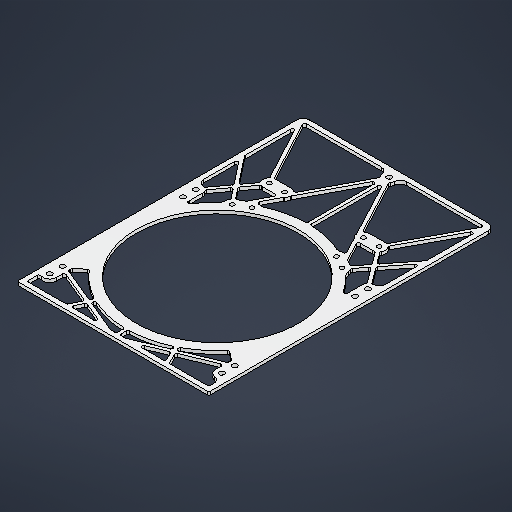
# Autodesk Inventor part: PLATE,SHOOTER,BOTTOM
Saved by Autodesk Inventor 2026.1 (Build 301233020, 233B)
## iProperties
Created: 2026-01-27
Part Number: PLATE,SHOOTER,BOTTOM
Material: Aluminum 6061
Document SubType Name: Sheet Metal
Designer: Owen L
Density: 2.7 g/cm^3
Appearance: Aluminum - Flat
Mass: 268.69 g
Surface Area: 679.811 cm^2
Volume: 99.5147 cm^3
Sheet Metal Rule: Default
Author: Owen L
Autodesk Inventor part; units mm, degrees
ref_plane "YZ Plane" through (0, 0, 0) normal (1, 0, 0) x (0, 1, 0)
ref_plane "XZ Plane" through (0, 0, 0) normal (0, 1, 0) x (-1, 0, 0)
ref_plane "XY Plane" through (0, 0, 0) normal (0, 0, 1) x (1, 0, 0)
sketch "Sketch1" plane through (0, 0, 0) normal (0, 1, 0) x (-1, 0, 0)
  line L0 (-93.6625, 139.7) -> (93.6625, 139.7)
  line L1 (93.6625, 139.7) -> (93.6625, -139.7)
  line L2 (93.6625, -139.7) -> (-93.6625, -139.7)
  line L3 (-93.6625, -139.7) -> (-93.6625, 139.7)
  line L4 (-93.6625, 139.7) -> (93.6625, -139.7) construction
  line L5 (93.6625, 139.7) -> (-93.6625, -139.7) construction
  circle A0 centre (0, 37.7949) radius 79.375
  point P0 (0, 0)
  dimension "d0" = 187.325
  dimension "d1" = 279.4
  dimension "d2" = 158.75
  dimension "d3" = 101.9051
  measures "d0" distance of L1.end L2.end
  measures "d1" distance of L0.end L1.end
  measures "d2" diameter of A0
  measures "d3" distance from line of L0 A0.centre
extrude "Plate1" add sketch "Sketch1" along normal blind 3.175
fillet "Corner Round1" radius 6.35 2 edges at (-93.6625, 1.5875, -139.7) (93.6625, 1.5875, -139.7)
fillet "Corner Round1" radius 1.5875 2 edges at (-93.6625, 1.5875, 139.7) (93.6625, 1.5875, 139.7)
sketch "Sketch2" plane through (0, 0, 0) normal (0, -1, 0) x (1, 0, 0)
  point P0 (0, 0)
  point P1 (-41.275, -37.3842)
  point P2 (-38.4175, -66.5942)
  point P3 (-53.6575, -66.5942)
  point P4 (-53.6575, -30.3992)
  dimension "d7" = 37.3842
  dimension "d11" = 41.275
  dimension "d12" = 6.985
  dimension "d13" = 29.21
  dimension "d14" = 2.8575
  dimension "d15" = 12.3825
  constraints: 1 horizontal alignment, 1 vertical alignment
  measures "d7" vertical distance of point (-41.275, -37.384) point (0, 0)
  measures "d11" horizontal distance of point (0, 0) point (-41.275, -37.384)
  measures "d12" vertical distance of point (-53.658, -30.399) point (-41.275, -37.384)
  measures "d13" vertical distance of point (-38.418, -66.594) point (-41.275, -37.384)
  measures "d14" horizontal distance of point (-38.418, -66.594) point (-41.275, -37.384)
  measures "d15" horizontal distance of point (-53.658, -66.594) point (-41.275, -37.384)
hole "Hole1" at (-41.275, 0, -37.3842) at (-38.4175, 0, -66.5942) at (-53.6575, 0, -66.5942) at (-53.6575, 0, -30.3992) direction (0, 1, 0) diameter 4.2926 depth 3.175 clearance for "Flat Head Machine Screw" size "M4" standard "Ansi Metric M Profile"
mirror "Mirror1" about plane through (0, 0, 0) normal (1, 0, 0) of "Hole1"
sketch "Sketch3" plane through (0, 3.175, 0) normal (0, 1, 0) x (1, 0, 0)
  line L0 (93.6625, -139.7) -> (-93.6625, -139.7) construction
  line L1 (93.6625, 133.35) -> (93.6625, -139.7) construction
  line L2 (-87.3125, 139.7) -> (87.3125, 139.7) construction
  line L3 (0, -139.7) -> (0, 139.7) construction
  point P0 (0, 0)
  point P1 (84.1375, -117.475)
  point P2 (84.1375, -104.775)
  point P3 (84.1375, 12.7)
  point P4 (84.1375, 25.4)
  point P5 (0, 130.175)
  point P6 (-84.1375, -117.475)
  point P7 (-84.1375, -104.775)
  point P8 (-84.1375, 12.7)
  point P9 (-84.1375, 25.4)
  dimension "d23" = 22.225
  dimension "d24" = 12.7
  dimension "d25" = 9.525
  dimension "d26" = 12.7
  dimension "d27" = 107.95
  dimension "d28" = 9.525
  constraints: 4 symmetric about line, 4 vertical alignment, 2 end point, 2 midpoint
  measures "d23" distance from line of L0 point (84.138, -117.475)
  measures "d24" distance of point (84.138, -104.775) point (84.138, -117.475)
  measures "d25" distance from line of L1 point (84.138, -117.475)
  measures "d26" distance of point (84.138, 25.4) point (84.138, 12.7)
  measures "d27" vertical distance of L1.start point (84.138, 25.4)
  measures "d28" distance from line of L2 point (0, 130.175)
hole "Hole2" at (84.1375, 3.175, 117.475) at (84.1375, 3.175, 104.775) at (84.1375, 3.175, -12.7) at (84.1375, 3.175, -25.4) at (0, 3.175, -130.175) at (-84.1375, 3.175, -25.4) at (-84.1375, 3.175, -12.7) at (-84.1375, 3.175, 104.775) at (-84.1375, 3.175, 117.475) direction (0, -1, 0) diameter 4.9784 depth 3.175 clearance for "Flat Head Machine Screw (82)" size "#10" standard "Ansi Unified Screw Threads"
sketch "Sketch4" plane through (0, 0, 0) normal (0, -1, 0) x (1, 0, 0)
  circle A0 centre (-84.1375, 117.475) radius 2.4892 projected
  circle A1 centre (-84.1375, 104.775) radius 2.4892 projected
  circle A2 centre (-84.1375, -12.7) radius 2.4892 projected
  circle A3 centre (-84.1375, -25.4) radius 2.4892 projected
  circle A4 centre (0, -130.175) radius 2.4892 projected
  circle A5 centre (84.1375, -25.4) radius 2.4892 projected
  circle A6 centre (84.1375, -12.7) radius 2.4892 projected
  circle A7 centre (84.1375, 104.775) radius 2.4892 projected
  circle A8 centre (84.1375, 117.475) radius 2.4892 projected
  circle A9 centre (53.6575, -30.3992) radius 2.1463 projected
  circle A10 centre (53.6575, -66.5942) radius 2.1463 projected
  circle A11 centre (38.4175, -66.5942) radius 2.1463 projected
  circle A12 centre (41.275, -37.3842) radius 2.1463 projected
  circle A13 centre (-53.6575, -30.3992) radius 2.1463 projected
  circle A14 centre (-53.6575, -66.5942) radius 2.1463 projected
  circle A15 centre (-38.4175, -66.5942) radius 2.1463 projected
  circle A16 centre (-41.275, -37.3842) radius 2.1463 projected
  circle A17 centre (0, 37.7949) radius 79.375 projected
  arc A18 (93.6625, 138.1125) -> (92.075, 139.7) centre (92.075, 138.1125) ccw projected
  line L0 (-92.075, 139.7) -> (92.075, 139.7) projected
  arc A19 (-92.075, 139.7) -> (-93.6625, 138.1125) centre (-92.075, 138.1125) ccw projected
  line L1 (-93.6625, -133.35) -> (-93.6625, 138.1125) projected
  arc A20 (-93.6625, -133.35) -> (-87.3125, -139.7) centre (-87.3125, -133.35) ccw projected
  line L2 (87.3125, -139.7) -> (-87.3125, -139.7) projected
  arc A21 (87.3125, -139.7) -> (93.6625, -133.35) centre (87.3125, -133.35) ccw projected
  line L3 (93.6625, 138.1125) -> (93.6625, -133.35) projected
  line L4 (-88.9, 134.9375) -> (88.9, 134.9375)
  line L5 (88.9, 134.9375) -> (88.9, -133.35)
  arc A22 (87.3125, -134.9375) -> (88.9, -133.35) centre (87.3125, -133.35) ccw
  line L6 (87.3125, -134.9375) -> (-87.3125, -134.9375)
  arc A23 (-88.9, -133.35) -> (-87.3125, -134.9375) centre (-87.3125, -133.35) ccw
  line L7 (-88.9, -133.35) -> (-88.9, 134.9375)
  circle A24 centre (0, 37.7949) radius 88.9
  circle A25 centre (0, -130.175) radius 6.35
  circle A26 centre (-84.1375, -25.4) radius 2.4892 projected
  circle A27 centre (-84.1375, -25.4) radius 6.35
  circle A28 centre (-84.1375, -12.7) radius 6.35
  circle A29 centre (-84.1375, 104.775) radius 6.35
  circle A30 centre (-84.1375, 117.475) radius 6.35
  circle A31 centre (84.1375, 104.775) radius 6.35
  circle A32 centre (84.1375, 117.475) radius 6.35
  circle A33 centre (84.1375, -12.7) radius 6.35
  circle A34 centre (84.1375, -25.4) radius 6.35
  circle A35 centre (-53.6575, -30.3992) radius 6.35
  circle A36 centre (-41.275, -37.3842) radius 6.35
  circle A37 centre (41.275, -37.3842) radius 6.35
  circle A38 centre (53.6575, -30.3992) radius 6.35
  circle A39 centre (38.4175, -66.5942) radius 6.35
  circle A40 centre (53.6575, -66.5942) radius 6.35
  circle A41 centre (-38.4175, -66.5942) radius 6.35
  circle A42 centre (-53.6575, -66.5942) radius 6.35
  line L8 (-77.7875, 117.475) -> (-77.7875, 104.775)
  line L9 (77.7875, 117.475) -> (77.7875, 104.775)
  line L10 (77.7875, -12.7) -> (77.7875, -25.4)
  line L11 (-77.7875, -25.4) -> (-77.7875, -12.7)
  line L12 (-56.7774, -35.9299) -> (-44.3949, -42.9149)
  line L13 (44.3949, -42.9149) -> (56.7774, -35.9299)
  line L14 (38.4175, -60.2442) -> (53.6575, -60.2442)
  line L15 (53.6575, -72.9442) -> (38.4175, -72.9442)
  line L16 (-53.6575, -60.2442) -> (-38.4175, -60.2442)
  line L17 (-38.4175, -72.9442) -> (-53.6575, -72.9442)
  arc A43 (-60.0071, -30.4684) -> (-56.7774, -35.9299) centre (-53.6575, -30.3992) ccw
  arc A44 (-60.0071, -30.4684) -> (-61.933, -25.9822) centre (-66.3567, -30.5377) ccw
  arc A45 (-44.3949, -42.9149) -> (-39.5612, -43.4986) centre (-41.275, -37.3842) ccw
  arc A46 (-35.3243, -43.7857) -> (-39.5612, -43.4986) centre (-37.8474, -49.6129) ccw
  arc A47 (39.5612, -43.4986) -> (44.3949, -42.9149) centre (41.275, -37.3842) ccw
  arc A48 (39.5612, -43.4986) -> (35.3243, -43.7857) centre (37.8474, -49.6129) ccw
  arc A49 (56.7774, -35.9299) -> (60.0071, -30.4684) centre (53.6575, -30.3992) ccw
  arc A50 (61.933, -25.9822) -> (60.0071, -30.4684) centre (66.3567, -30.5377) ccw
  arc A51 (77.7875, -25.4) -> (83.3438, -31.7002) centre (84.1375, -25.4) ccw
  arc A52 (88.9, -38.0004) -> (83.3438, -31.7002) centre (82.55, -38.0004) ccw
  line L18 (0, -123.825) -> (12.1384, -123.825) construction
  line L19 (0, -123.825) -> (-9.725, -123.825) construction
  arc A53 (0, -123.825) -> (-6.3002, -129.3813) centre (0, -130.175) ccw
  arc A54 (-12.6004, -134.9375) -> (-6.3002, -129.3813) centre (-12.6004, -128.5875) ccw
  arc A55 (6.3002, -129.3813) -> (0, -123.825) centre (0, -130.175) ccw
  arc A56 (6.3002, -129.3813) -> (12.6004, -134.9375) centre (12.6004, -128.5875) ccw
  arc A57 (-83.3438, -31.7002) -> (-77.7875, -25.4) centre (-84.1375, -25.4) ccw
  arc A58 (-83.3438, -31.7002) -> (-88.9, -38.0004) centre (-82.55, -38.0004) ccw
  arc A59 (-83.3438, 98.4748) -> (-77.7875, 104.775) centre (-84.1375, 104.775) ccw
  arc A60 (-83.3438, 98.4748) -> (-88.9, 92.1746) centre (-82.55, 92.1746) ccw
  arc A61 (-77.7875, 117.475) -> (-83.3438, 123.7752) centre (-84.1375, 117.475) ccw
  arc A62 (83.3438, 123.7752) -> (77.7875, 117.475) centre (84.1375, 117.475) ccw
  arc A63 (83.3438, 123.7752) -> (88.9, 130.0754) centre (82.55, 130.0754) ccw
  arc A64 (77.7875, 104.775) -> (83.3438, 98.4748) centre (84.1375, 104.775) ccw
  arc A65 (88.9, 92.1746) -> (83.3438, 98.4748) centre (82.55, 92.1746) ccw
  arc A66 (-88.9, 130.0754) -> (-83.3438, 123.7752) centre (-82.55, 130.0754) ccw
  line L20 (-84.1375, 104.775) -> (0, 139.7) construction
  line L21 (-83.5289, 103.3088) -> (0.6086, 138.2338)
  line L22 (-0.6086, 141.1662) -> (-84.7461, 106.2412)
  arc A67 (-84.7461, 106.2412) -> (-83.5289, 103.3088) centre (-84.1375, 104.775) ccw
  arc A68 (0.6086, 138.2338) -> (-0.6086, 141.1662) centre (0, 139.7) ccw
  line L23 (0, 139.7) -> (84.1375, 104.775) construction
  line L24 (-0.6086, 138.2338) -> (83.5289, 103.3088)
  line L25 (84.7461, 106.2412) -> (0.6086, 141.1662)
  arc A69 (0.6086, 141.1662) -> (-0.6086, 138.2338) centre (0, 139.7) ccw
  arc A70 (83.5289, 103.3088) -> (84.7461, 106.2412) centre (84.1375, 104.775) ccw
  line L26 (0, 139.7) -> (0, -139.7) construction
  line L27 (-1.5875, 139.7) -> (-1.5875, -139.7)
  line L28 (1.5875, -139.7) -> (1.5875, 139.7)
  arc A71 (1.5875, 139.7) -> (-1.5875, 139.7) centre (0, 139.7) ccw
  arc A72 (-1.5875, -139.7) -> (1.5875, -139.7) centre (0, -139.7) ccw
  line L29 (0, -130.175) -> (-88.9, 37.7949) construction
  line L30 (1.4031, -129.4324) -> (-87.4969, 38.5376)
  line L31 (-90.3031, 37.0523) -> (-1.4031, -130.9176)
  arc A73 (-1.4031, -130.9176) -> (1.4031, -129.4324) centre (0, -130.175) ccw
  arc A74 (-87.4969, 38.5376) -> (-90.3031, 37.0523) centre (-88.9, 37.7949) ccw
  line L32 (0, -130.175) -> (88.9, 37.7949) construction
  line L33 (1.4031, -130.9176) -> (90.3031, 37.0523)
  line L34 (87.4969, 38.5376) -> (-1.4031, -129.4324)
  arc A75 (-1.4031, -129.4324) -> (1.4031, -130.9176) centre (0, -130.175) ccw
  arc A76 (90.3031, 37.0523) -> (87.4969, 38.5376) centre (88.9, 37.7949) ccw
  line L35 (-53.6575, -66.5942) -> (-91.8026, -137.8401) construction
  line L36 (-55.057, -65.8449) -> (-93.2022, -137.0908)
  line L37 (-90.4031, -138.5894) -> (-52.258, -67.3435)
  arc A77 (-52.258, -67.3435) -> (-55.057, -65.8449) centre (-53.6575, -66.5942) ccw
  arc A78 (-93.2022, -137.0908) -> (-90.4031, -138.5894) centre (-91.8026, -137.8401) ccw
  line L38 (53.6575, -66.5942) -> (91.8026, -137.8401) construction
  line L39 (52.258, -67.3435) -> (90.4031, -138.5894)
  line L40 (93.2022, -137.0908) -> (55.057, -65.8449)
  arc A79 (55.057, -65.8449) -> (52.258, -67.3435) centre (53.6575, -66.5942) ccw
  arc A80 (90.4031, -138.5894) -> (93.2022, -137.0908) centre (91.8026, -137.8401) ccw
  line L41 (-53.6575, -66.5942) -> (-84.1375, -25.4) construction
  line L42 (-52.3813, -65.65) -> (-82.8613, -24.4558)
  line L43 (-85.4137, -26.3442) -> (-54.9337, -67.5384)
  arc A81 (-54.9337, -67.5384) -> (-52.3813, -65.65) centre (-53.6575, -66.5942) ccw
  arc A82 (-82.8613, -24.4558) -> (-85.4137, -26.3442) centre (-84.1375, -25.4) ccw
  line L44 (53.6575, -66.5942) -> (84.1375, -25.4) construction
  line L45 (54.9337, -67.5384) -> (85.4137, -26.3442)
  line L46 (82.8613, -24.4558) -> (52.3813, -65.65)
  arc A83 (52.3813, -65.65) -> (54.9337, -67.5384) centre (53.6575, -66.5942) ccw
  arc A84 (85.4137, -26.3442) -> (82.8613, -24.4558) centre (84.1375, -25.4) ccw
  line L47 (0, 37.7949) -> (-93.6625, -81.2422) construction
  line L48 (-93.6625, 138.1125) -> (-93.6625, -133.35) projected
  line L49 (-1.2476, 38.7766) -> (-94.9101, -80.2605)
  line L50 (-92.4149, -82.2238) -> (1.2476, 36.8133)
  arc A85 (1.2476, 36.8133) -> (-1.2476, 38.7766) centre (0, 37.7949) ccw
  arc A86 (-94.9101, -80.2605) -> (-92.4149, -82.2238) centre (-93.6625, -81.2422) ccw
  line L51 (0, 37.7949) -> (93.6625, -81.2422) construction
  line L52 (-1.2476, 36.8133) -> (92.4149, -82.2238)
  line L53 (94.9101, -80.2605) -> (1.2476, 38.7766)
  arc A87 (1.2476, 38.7766) -> (-1.2476, 36.8133) centre (0, 37.7949) ccw
  arc A88 (92.4149, -82.2238) -> (94.9101, -80.2605) centre (93.6625, -81.2422) ccw
  line L54 (0, 37.7949) -> (50.7685, 139.7) construction
  line L55 (1.4209, 37.087) -> (52.1894, 138.9921)
  line L56 (49.3475, 140.4079) -> (-1.4209, 38.5028)
  arc A89 (-1.4209, 38.5028) -> (1.4209, 37.087) centre (0, 37.7949) ccw
  arc A90 (52.1894, 138.9921) -> (49.3475, 140.4079) centre (50.7685, 139.7) ccw
  line L57 (0, 37.7949) -> (-50.7685, 139.7) construction
  line L58 (1.4209, 38.5028) -> (-49.3475, 140.4079)
  line L59 (-52.1894, 138.9921) -> (-1.4209, 37.087)
  arc A91 (-1.4209, 37.087) -> (1.4209, 38.5028) centre (0, 37.7949) ccw
  arc A92 (-49.3475, 140.4079) -> (-52.1894, 138.9921) centre (-50.7685, 139.7) ccw
  line L60 (0, 37.7949) -> (-84.1375, -12.7) construction
  line L61 (-0.8169, 39.1561) -> (-84.9544, -11.3388)
  line L62 (-83.3206, -14.0612) -> (0.8169, 36.4338)
  arc A93 (0.8169, 36.4338) -> (-0.8169, 39.1561) centre (0, 37.7949) ccw
  arc A94 (-84.9544, -11.3388) -> (-83.3206, -14.0612) centre (-84.1375, -12.7) ccw
  line L63 (0, 37.7949) -> (84.1375, -12.7) construction
  line L64 (-0.8169, 36.4338) -> (83.3206, -14.0612)
  line L65 (84.9544, -11.3388) -> (0.8169, 39.1561)
  arc A95 (0.8169, 39.1561) -> (-0.8169, 36.4338) centre (0, 37.7949) ccw
  arc A96 (83.3206, -14.0612) -> (84.9544, -11.3388) centre (84.1375, -12.7) ccw
  line L66 (0, 37.7949) -> (-84.1375, 104.775) construction
  line L67 (0.9887, 39.0369) -> (-83.1488, 106.017)
  line L68 (-85.1262, 103.533) -> (-0.9887, 36.5529)
  arc A97 (-0.9887, 36.5529) -> (0.9887, 39.0369) centre (0, 37.7949) ccw
  arc A98 (-83.1488, 106.017) -> (-85.1262, 103.533) centre (-84.1375, 104.775) ccw
  line L69 (0, 37.7949) -> (84.1375, 104.775) construction
  line L70 (0.9887, 36.5529) -> (85.1262, 103.533)
  line L71 (83.1488, 106.017) -> (-0.9887, 39.0369)
  arc A99 (-0.9887, 39.0369) -> (0.9887, 36.5529) centre (0, 37.7949) ccw
  arc A100 (85.1262, 103.533) -> (83.1488, 106.017) centre (84.1375, 104.775) ccw
  point P0 (0, 0)
  point P1 (-42.0687, 122.2375)
  point P2 (42.0688, 122.2375)
  point P3 (0, 0)
  point P4 (-44.45, -46.19)
  point P5 (44.45, -46.19)
  point P6 (-72.7301, -102.2172)
  point P7 (72.7301, -102.2172)
  point P8 (-68.8975, -45.9971)
  point P9 (68.8975, -45.9971)
  point P10 (-46.8313, -21.7236)
  point P11 (46.8313, -21.7236)
  point P12 (25.3842, 88.7475)
  point P13 (-25.3842, 88.7475)
  point P14 (-42.0688, 12.5475)
  point P15 (42.0688, 12.5475)
  point P16 (-42.0687, 71.285)
  point P17 (42.0688, 71.285)
  point P18 (-79.2043, -29.3983)
  point P19 (-67.4208, -45.3239)
  point P20 (-58.707, -34.2495)
  point P21 (-75.3971, -9.3059)
  point P22 (-78.0488, -10.8973)
  point P23 (-88.9, -72.6222)
  point P24 (-69.4563, -47.9109)
  point P25 (-81.7566, -31.2868)
  point P26 (-83.3438, -31.7002)
  point P27 (-67.4984, -50.557)
  point P28 (-88.9, -77.7567)
  point P29 (-88.9, -129.0554)
  point P30 (-57.9591, -71.2653)
  point P31 (-58.5907, -62.5959)
  point P32 (-56.2315, -36.2378)
  point P33 (-65.4629, -47.9701)
  point P34 (-56.0384, -60.7074)
  point P35 (-38.8016, -60.2558)
  point P36 (-49.5053, -40.0321)
  point P37 (-55.16, -72.7639)
  point P38 (-88.2742, -134.6131)
  point P39 (-4.2792, -125.4834)
  point P40 (-33.3924, -70.4763)
  point P41 (-44.384, -42.921)
  point P42 (-1.5875, -123.7819)
  point P43 (-1.5875, -51.0909)
  point P44 (88.2742, -134.6131)
  point P45 (55.16, -72.7639)
  point P46 (33.3924, -70.4763)
  point P47 (4.2792, -125.4834)
  point P48 (6.3002, -129.3813)
  point P49 (1.5875, -123.7819)
  point P50 (44.384, -42.921)
  point P51 (39.5612, -43.4986)
  point P52 (1.5875, -51.0909)
  point P53 (88.9, -77.7567)
  point P54 (67.4984, -50.557)
  point P55 (58.5907, -62.5959)
  point P56 (57.9591, -71.2653)
  point P57 (88.9, -129.0554)
  point P58 (65.4629, -47.9701)
  point P59 (56.2315, -36.2378)
  point P60 (49.5053, -40.0321)
  point P61 (38.8016, -60.2558)
  point P62 (56.0384, -60.7074)
  point P63 (69.4563, -47.9109)
  point P64 (88.9, -72.6222)
  point P65 (83.3438, -31.7002)
  point P66 (81.7566, -31.2868)
  point P67 (78.0488, -10.8973)
  point P68 (75.3971, -9.3059)
  point P69 (60.0071, -30.4684)
  point P70 (58.707, -34.2495)
  point P71 (67.4208, -45.3239)
  point P72 (79.2043, -29.3983)
  point P73 (68.5523, 94.397)
  point P74 (78.3385, 102.1877)
  point P75 (77.7875, 105.692)
  point P76 (42.8288, 120.2032)
  point P77 (41.0569, 116.6463)
  point P78 (50.1694, 134.9375)
  point P79 (44.248, 123.0517)
  point P80 (77.7875, 109.1297)
  point P81 (41.3087, 124.2718)
  point P82 (46.6222, 134.9375)
  point P83 (15.6141, 134.9375)
  point P84 (38.215, 118.0621)
  point P85 (39.8895, 121.4233)
  point P86 (7.3325, 134.9375)
  point P87 (1.5875, 134.9375)
  point P88 (1.5875, 126.6808)
  point P89 (-46.6222, 134.9375)
  point P90 (-41.3087, 124.2718)
  point P91 (-15.6141, 134.9375)
  point P92 (-39.8895, 121.4233)
  point P93 (-38.215, 118.0621)
  point P94 (-1.5875, 126.6808)
  point P95 (-1.5875, 134.9375)
  point P96 (-7.3325, 134.9375)
  point P97 (-78.3385, 102.1877)
  point P98 (-68.5523, 94.397)
  point P99 (-41.0569, 116.6463)
  point P100 (-42.8288, 120.2032)
  point P101 (-77.7875, 105.692)
  point P102 (-44.248, 123.0517)
  point P103 (-50.1694, 134.9375)
  point P104 (-88.9, 121.6751)
  point P105 (-77.7875, 109.1297)
  point P106 (-52.8878, -26.8537)
  point P107 (-51.2631, -29.9234)
  point P108 (-55.0355, -29.5832)
  point P109 (-38.8078, -60.2442)
  point P110 (-32.082, -66.1647)
  point P111 (-53.4108, -32.6529)
  point P112 (-34.4996, -61.597)
  point P113 (52.8878, -26.8537)
  point P114 (55.0355, -29.5832)
  point P115 (32.082, -66.1647)
  point P116 (51.2631, -29.9234)
  point P117 (34.4996, -61.597)
  point P118 (38.8078, -60.2442)
  point P119 (53.4108, -32.6529)
  point P120 (56.2118, -36.2128)
  point P121 (-56.2118, -36.2128)
  dimension "d38" = 12.7
  dimension "d37" = 4.7625
  dimension "d39" = 6.35
  dimension "d40" = 3.175
  dimension "d41" = 3.175
  dimension "d42" = 3.175
  dimension "d43" = 3.175
  dimension "d44" = 3.175
  dimension "d45" = 3.175
  dimension "d46" = 3.175
  dimension "d47" = 3.175
  dimension "d48" = 3.175
  dimension "d49" = 3.175
  dimension "d50" = 3.175
  dimension "d51" = 3.175
  dimension "d52" = 3.175
  dimension "d53" = 3.175
  dimension "d54" = 3.175
  dimension "d55" = 3.175
  dimension "d56" = 3.175
  constraints: 168 end point, 136 point on circle, 95 tangent, 65 centre point, 35 equal radius, 26 point on line, 19 midpoint, 19 parallel, 17 coincident, 4 horizontal, 3 vertical, 1 concentric, 52 other
  measures "d37" distance between parallel lines of L1 L7
  measures "d39" radius of A54
  measures "d40" diameter of A68
  measures "d41" diameter of A70
  measures "d42" diameter of A72
  measures "d43" diameter of A74
  measures "d44" diameter of A76
  measures "d45" diameter of A78
  measures "d46" diameter of A80
  measures "d47" diameter of A82
  measures "d48" diameter of A84
  measures "d49" diameter of A86
  measures "d50" diameter of A88
  measures "d51" diameter of A90
  measures "d52" diameter of A92
  measures "d53" diameter of A94
  measures "d54" diameter of A96
  measures "d55" diameter of A98
  measures "d56" diameter of A100
extrude "Cut1" cut sketch "Sketch4" against normal blind 3.175 contours A29 L8 L21 L59 A24 L67 | L8 A30 A66 L7 L4 L59 L22 | L7 A66 A30 | L58 L4 L22 | L21 L4 L27 A24 L58 | L28 L4 L24 L56 A24 | A24 A44 A35 L49 L42 A27 L11 A28 L62 | L55 L24 L9 A31 L71 A24 | L4 L56 L25 | L7 A58 A27 L43 L49 | L55 L4 L5 A63 A32 L9 L25 | L27 L30 A41 A36 A46 A24 | L50 L43 A42 L36 L7 | A24 A48 A37 L34 A39 L28 | L50 L12 L31 L16 A42 L42 | A25 A54 L6 A23 L37 A42 L17 A41 L31 | L36 L43 A81 L37 A14 | A14 L43 L36 | A14 L42 A77 L36 L43 | A14 L37 A77 L42 | L33 A39 L15 A40 L39 A22 L6 A56 A25 | L53 L45 A34 A52 L5 | L36 A77 A81 L43 | L64 A33 L10 A34 L46 L53 A38 A50 A24 | L5 L40 A40 L45 L52 | L13 L52 L46 A40 L14 L33 | L39 A83 L45 L40 A10 | A10 L46 A79 L39 | L40 L45 A10 | L45 L40 A79 L46 A10 | A79 L40 L45 A83 | A11 | A15
fillet "Corner Round2" radius 1.5875 89 edges at (-55.16, 1.5875, -72.7639) (-88.2742, 1.5875, -134.6131) (-88.9, 1.5875, -72.6222) (-33.3924, 1.5875, -70.4763) (-69.4563, 1.5875, -47.9109) (-67.4984, 1.5875, -50.557) (-58.5907, 1.5875, -62.5959) (-57.9591, 1.5875, -71.2653) (-81.7566, 1.5875, -31.2868) (-79.2043, 1.5875, -29.3983) (-67.4208, 1.5875, -45.3239) (-75.3971, 1.5875, -9.3059) (-78.0488, 1.5875, -10.8973) (-58.707, 1.5875, -34.2495) (-56.0384, 1.5875, -60.7074) (58.707, 1.5875, -34.2495) (67.4208, 1.5875, -45.3239) (88.9, 1.5875, -129.0554) (88.2742, 1.5875, -134.6131) (79.2043, 1.5875, -29.3983) (75.3971, 1.5875, -9.3059) (78.0488, 1.5875, -10.8973) (56.2315, 1.5875, -36.2378) (49.5053, 1.5875, -40.0321) (56.0384, 1.5875, -60.7074) (-44.384, 1.5875, -42.921) (58.5907, 1.5875, -62.5959) (57.9591, 1.5875, -71.2653) (33.3924, 1.5875, -70.4763) (88.9, 1.5875, -72.6222) (81.7566, 1.5875, -31.2868) (69.4563, 1.5875, -47.9109) (65.4629, 1.5875, -47.9701) (-88.9, 1.5875, -77.7567) (4.2792, 1.5875, -125.4834) (-1.5875, 1.5875, -123.7819) (-88.9, 1.5875, -129.0554) (-1.5875, 1.5875, -51.0909) (-65.4629, 1.5875, -47.9701) (-56.2315, 1.5875, -36.2378) (44.384, 1.5875, -42.921) (1.5875, 1.5875, -51.0909) (1.5875, 1.5875, -123.7819) (67.4984, 1.5875, -50.557) (-4.2792, 1.5875, -125.4834) (55.16, 1.5875, -72.7639) (88.9, 1.5875, -77.7567) (-44.248, 1.5875, 123.0517) (-77.7875, 1.5875, 109.1297) (39.8895, 1.5875, 121.4233) (-50.1694, 1.5875, 134.9375) (78.3385, 1.5875, 102.1877) (38.215, 1.5875, 118.0621) (42.8288, 1.5875, 120.2032) (1.5875, 1.5875, 126.6808) (-88.9, 1.5875, 121.6751) (-88.9, 1.5875, 134.9375) (-68.5523, 1.5875, 94.397) (7.3325, 1.5875, 134.9375) (1.5875, 1.5875, 134.9375) (68.5523, 1.5875, 94.397) (41.0569, 1.5875, 116.6463) (46.6222, 1.5875, 134.9375) (-41.0569, 1.5875, 116.6463) (-77.7875, 1.5875, 105.692) (-15.6141, 1.5875, 134.9375) (-46.6222, 1.5875, 134.9375) (-42.8288, 1.5875, 120.2032) (-78.3385, 1.5875, 102.1877) (-41.3087, 1.5875, 124.2718) (77.7875, 1.5875, 105.692) (-38.215, 1.5875, 118.0621) (-39.8895, 1.5875, 121.4233) (77.7875, 1.5875, 109.1297) (-7.3325, 1.5875, 134.9375) (-1.5875, 1.5875, 126.6808) (-1.5875, 1.5875, 134.9375) (50.1694, 1.5875, 134.9375) (88.9, 1.5875, 134.9375) (44.248, 1.5875, 123.0517) (15.6141, 1.5875, 134.9375) (41.3087, 1.5875, 124.2718) (-49.5053, 1.5875, -40.0321) (38.8078, 1.5875, -60.2442) (32.082, 1.5875, -66.1647) (34.4996, 1.5875, -61.597) (-38.8078, 1.5875, -60.2442) (-34.4996, 1.5875, -61.597) (-32.082, 1.5875, -66.1647)
equation "\"d21\" = Thickness"
equation "\"d34\" = Thickness"
equation "\"d57\" = Thickness"
equation "\"d4\" = Thickness"
equation "\"BendRadius\" = Thickness"
equation "\"BendReliefWidth\" = Thickness"
equation "\"BendReliefDepth\" = 0.5 * Thickness"
equation "\"CornerReliefSize\" = 4 * Thickness"
equation "\"MinimumRemnant\" = 2 * Thickness"
equation "\"TransitionRadius\" = BendRadius"
equation "\"JacobiRadiusSize\" = BendRadius"
equation "\"GapSize\" = Thickness"
equation "\"Thickness\" = 3.175"
body "Solid1"
